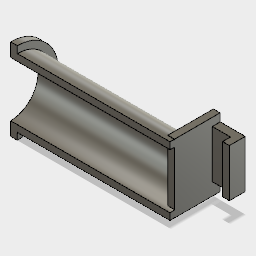
手机支架 v1 (Autodesk Fusion 360 design; units mm, degrees)
Autodesk Fusion 360 part; units mm, degrees
sketch "草图1" plane through (0, 0, 0) normal (0, 1, 0) x (1, 0, 0)
  line L0 (30, -20) -> (41, -20)
  line L1 (41, -20) -> (44, -20)
  line L2 (44, -20) -> (44, -40)
  line L3 (44, -40) -> (41, -40)
  line L4 (41, -40) -> (41, -20)
  line L5 (30, -20) -> (30, -27)
  line L6 (30, -27) -> (33, -27)
  line L7 (33, -27) -> (33, -23.5)
  line L8 (33, -23.5) -> (41, -23.5)
extrude "拉伸1" add sketch "草图1" along normal blind 21 contours L0 L4 L5 L6 L7 L8 makes body 1
move_body "移动1" bodies 1 to x (1, 0, 0) y (0, 1, 0) z (0, 0, 1) at (-5, 0, 0)
extrude "拉伸2" add sketch "草图1" along normal blind 30 separate body contours L1 L2 L3 L4 makes body 2
sketch "草图2" plane through (0, 0, 0) normal (0, 1, 0) x (1, 0, 0)
sketch "草图3" plane through (0, 0, 0) normal (0, 1, 0) x (1, 0, 0)
  arc A0 (45, -10) -> (15, -10) centre (30, -10) ccw
  arc A1 (48, -10) -> (12, -10) centre (30, -10) ccw
  arc A2 (42, -10) -> (18, -10) centre (30, -10) ccw
  line L0 (12, -10) -> (15, -10)
  line L1 (18, -10) -> (15, -10)
  line L2 (42, -10) -> (45, -10)
  line L3 (45, -10) -> (48, -10)
  dimension "d7" = 3
  dimension "d8" = 3
extrude "拉伸3" add sketch "草图3" along normal blind 70 separate body contours A0 A2 L1 L2 makes body 3
extrude "拉伸4" add sketch "草图3" along normal blind 3 contours A0 A1 L0 L3 bodies 3
move_body "移动2" bodies 3 to x (0, -1, 0) y (1, 0, 0) z (0, 0, 1) at (57.8229, 58.0226, -12.9298)
move_body "对齐1" bodies 3 to x (1, 0, 0) y (0, 1, 0) z (0, 0, 1) at (-16.8229, 0, 0)
move_body "移动3" bodies 2 to x (1, 0, 0) y (0, 1, 0) z (0, 0, 1) at (76.8079, 8.1463, 0)
move_body "对齐2" bodies 3 to x (1, 0, 0) y (0, 1, 0) z (0, 0, 1) at (9.8079, -4.8763, 44.9298)
move_body "移动4" bodies 1 to x (-1, 0, 0) y (0, -1, 0) z (0, 0, 1) at (165.9741, 30.1646, 0)
move_body "移动5" bodies 1 to x (1, 0, 0) y (0, 1, 0) z (0, 0, 1) at (26.0813, 15.5062, -20.369)
move_body "对齐3" bodies 1 to x (1, 0, 0) y (0, 0, -1) z (0, 1, 0) at (-35.2475, 21.7653, 75.1707)
move_body "移动6" bodies 1 to x (1, 0, 0) y (0, 0, 1) z (0, -1, 0) at (0, 71.8963, 29.1037)
move_body "移动7" bodies 1 to x (1, 0, 0) y (0, 1, 0) z (0, 0, 1) at (0.1041, -7.615, -30.4398)
combine "合并1" operation add target body 1 tool bodies 2 3 makes body 4 at (75.1412, 23.1463, 27)
